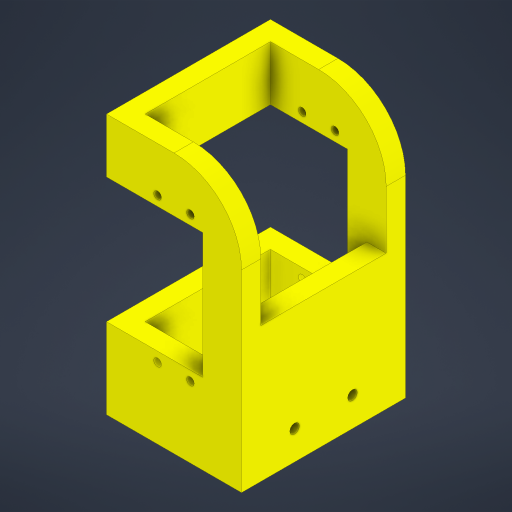
# Autodesk Inventor part: Joint_3_House
Saved by Autodesk Inventor 2023 (Build 270158000, 158)
## iProperties
Created: 2023-08-18
Part Number: Joint_3_House
Material: Acrylic, Clear
Document SubType Name: Modeling
Designer: Abhinav
Density: 1.19 g/cm^3
Appearance: Default(1)
Mass: 222.964 g
Surface Area: 490.764 cm^2
Volume: 187.364 cm^3
Author: Abhinav
Autodesk Inventor part; units mm, degrees
ref_plane "YZ Plane" through (0, 0, 0) normal (1, 0, 0) x (0, 1, 0)
ref_plane "XZ Plane" through (0, 0, 0) normal (0, 1, 0) x (-1, 0, 0)
sketch "Sketch1" plane through (0, 0, 0) normal (0, 0, 1) x (1, 0, 0)
  line L0 (0, 37.5) -> (8.5, 37.5) construction
  circle A0 centre (8.5, 37.5) radius 2
  line L1 (8.5, 37.5) -> (-8.5, 37.5) construction
  line L2 (-8.5, 37.5) -> (-8.5, -37.5) construction
  line L3 (-8.5, -37.5) -> (8.5, -37.5) construction
  line L4 (8.5, -37.5) -> (8.5, 37.5) construction
  circle A1 centre (8.5, -37.5) radius 2
  line L5 (-8.5, 37.5) -> (8.5, -37.5) construction
  line L6 (-14.9, 32.5) -> (14.9, 32.5)
  line L7 (14.9, 32.5) -> (14.9, -32.5)
  line L8 (14.9, -32.5) -> (-14.9, -32.5)
  line L9 (-14.9, 32.5) -> (14.9, -32.5) construction
  line L10 (14.9, 32.5) -> (-14.9, -32.5) construction
  circle A2 centre (-8.5, -37.5) radius 2
  circle A3 centre (-8.5, 37.5) radius 2
  arc A4 (-8.5, -20) -> (-9.1777, -20.0184) centre (-8.5, -32.5) ccw
  line L11 (0, 19) -> (0, 0) construction
  line L12 (0, 32.5) -> (0, 19) construction
  line L13 (35, 25.75) -> (35, -74.25)
  line L14 (35, -74.25) -> (-35, -74.25)
  line L15 (-35, -74.25) -> (-35, -32.5)
  arc A5 (35, 25.75) -> (0, 60.75) centre (0, 25.75) ccw
  line L16 (0, 60.75) -> (-35, 60.75)
  line L17 (-35, 60.75) -> (-35, 32.5)
  line L18 (-14.9, -32.5) -> (-35, -32.5)
  line L19 (-14.9, 32.5) -> (-35, 32.5)
  point P0 (8.5, -32.5)
  dimension "d0" = 8.5
  dimension "d1" = 4
  dimension "d2" = 17
  dimension "d3" = 75
  dimension "d4" = 4
  dimension "d5" = 29.8
  dimension "d6" = 65
  dimension "d7" = 4
  dimension "d8" = 4
  dimension "d9" = 13.5
  dimension "d12" = 100
  dimension "d15" = 35
  constraints: 40 end point, 6 centre point, 5 midpoint, 5 perpendicular, 4 coincident, 4 parallel, 4 point on circle, 4 point on line, 3 horizontal, 2 tangent, 1 symmetric about line, 1 vertical
  measures "d0" distance of L0.start L0.end
  measures "d1" diameter of A0
  measures "d2" distance of L4.start L2.end
  measures "d3" distance of L2.end L2.start
  measures "d4" diameter of A1
  measures "d5" distance of L7.end L10.end
  measures "d6" distance of L7.start L7.end
  measures "d7" diameter of A2
  measures "d8" diameter of A3
  measures "d9" distance of L12.start L11.start
  measures "d12" distance of L13.start L13.end
  measures "d15" radius of A5
extrude "Extrusion1" add sketch "Sketch1" along normal blind 10
ref_plane "Work Plane1" through (0, 0, -65) normal (0, 0, -1) x (-1, 0, 0)
sketch "Sketch2" plane through (0, 0, -65) normal (0, 0, -1) x (-1, 0, 0)
  line L0 (35, -32.5) -> (35, -74.25) projected
  arc A0 (0, 60.75) -> (-35, 25.75) centre (0, 25.75) ccw projected
  line L1 (-35, -74.25) -> (-35, 25.75) projected
  line L2 (35, -74.25) -> (-35, -74.25) projected
  circle A1 centre (-8.5, -37.5) radius 2 projected
  circle A2 centre (8.5, -37.5) radius 2 projected
  circle A3 centre (8.5, 37.5) radius 2 projected
  circle A4 centre (-8.5, 37.5) radius 2 projected
  line L3 (-14.9, 32.5) -> (-14.9, -32.5) projected
  line L4 (35, 32.5) -> (-14.9, 32.5) projected
  line L5 (-14.9, -32.5) -> (35, -32.5) projected
  line L6 (35, 60.75) -> (35, 32.5) projected
  line L7 (0, 60.75) -> (35, 60.75) projected
  point P0 (0, 0)
extrude "Extrusion2" add sketch "Sketch2" along normal blind 10
sketch "Sketch3" plane through (0, 0, 0) normal (0, 0, -1) x (-1, 0, 0)
  line L0 (-35, -74.25) -> (-35, 25.75) projected
  line L1 (-35, -74.25) -> (-25, -74.25)
  line L2 (-25, -74.25) -> (-25, -4.25)
  line L3 (-25, -4.25) -> (-35, -4.25)
  line L4 (-35, -4.25) -> (-35, -74.25)
  line L5 (35, -74.25) -> (-35, -74.25) projected
  line L6 (-14.9, -32.5) -> (35, -32.5) projected
  line L7 (35, -74.25) -> (25, -74.25)
  line L8 (25, -74.25) -> (25, -32.5)
  line L9 (25, -32.5) -> (35, -32.5)
  line L10 (35, -32.5) -> (35, -74.25)
  line L11 (35, 60.75) -> (35, 32.5) projected
  line L12 (35, 32.5) -> (-14.9, 32.5) projected
  line L13 (35, 60.75) -> (25, 60.75)
  line L14 (25, 60.75) -> (25, 32.5)
  line L15 (25, 32.5) -> (35, 32.5)
  line L16 (35, 32.5) -> (35, 60.75)
  point P0 (0, 0)
  point P1 (-35, -4.25)
  dimension "d19" = 10
  dimension "d23" = 70
  dimension "d24" = 10
  dimension "d25" = 10
  constraints: 24 end point, 6 parallel, 3 horizontal, 3 perpendicular, 2 point on line
  measures "d19" distance of L3.end L2.end
  measures "d23" distance of L3.end L0.start
  measures "d24" distance of L8.end L9.end
  measures "d25" distance of L15.end L14.end
extrude "Extrusion3" add sketch "Sketch3" along normal up to next
sketch "Sketch4" plane through (35, 0, 10) normal (1, 0, 0) x (0, 0, -1)
  line L0 (85, 25.75) -> (85, -74.25) projected
  line L1 (0, -32.5) -> (0, -74.25) projected
  line L2 (85, -74.25) -> (0, -74.25)
  line L3 (0, -74.25) -> (0, -44.25)
  line L4 (0, -44.25) -> (85, -44.25)
  line L5 (85, -44.25) -> (85, -74.25)
  line L6 (0, -74.25) -> (85, -74.25) construction
  line L7 (85, -44.25) -> (0, -74.25) construction
  line L8 (42.5, -59.25) -> (57.5, -59.25) construction
  line L9 (42.5, -59.25) -> (27.5, -59.25) construction
  circle A0 centre (57.5, -59.25) radius 2.5
  circle A1 centre (27.5, -59.25) radius 2.5
  point P0 (10, 0)
  dimension "d26" = 30
  dimension "d27" = 15
  dimension "d28" = 15
  dimension "d29" = 5
  dimension "d30" = 5
  constraints: 14 end point, 3 horizontal, 2 centre point, 2 coincident, 2 parallel, 1 midpoint, 1 perpendicular, 1 point on line
  measures "d26" distance of L2.end L3.end
  measures "d27" distance of L8.start L8.end
  measures "d28" distance of L8.start L9.end
  measures "d29" diameter of A0
  measures "d30" diameter of A1
extrude "Extrusion4" cut sketch "Sketch4" against normal blind 90 contours A0 | A1
body "Solid1"
